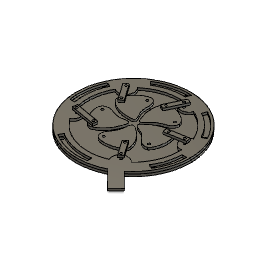
Final Design Machine_Lab v3 (Autodesk Fusion 360 design; units mm, degrees)
Autodesk Fusion 360 part; units mm, degrees
note: some values were not read from the file. Chosen so that the rebuilt part matches the saved one: which face or edge a step refers to; which pieces of a blend or face edit are solid. Set by a fixed rule: which sketch regions a step uses.
sketch "Sketch1" plane through (0, 0, 0) normal (0, 1, 0) x (1, 0, 0)
  spline S0 degree 5 poles (43.1472, 9.785) (42.8335, 10.0513) (42.2447, 10.6075) (41.4786, 11.5091) (40.6873, 12.8271) (40.039, 14.6039) (39.669, 16.4398) (39.5104, 18.2683) (39.5055, 20.0358) (39.6219, 21.7131) (39.8483, 23.293) (40.1848, 24.7857) (40.6367, 26.2147) (41.2054, 27.6126) (41.8835, 29.017) (42.6573, 30.4642) (43.5081, 31.9837) (44.4141, 33.5928) (45.3515, 35.2894) (46.2961, 37.0569) (47.2231, 38.8737) (48.108, 40.7214) (48.9268, 42.5931) (49.6569, 44.5023) (50.2774, 46.4894) (50.7734, 48.6052) (51.1395, 50.8969) (51.3829, 53.3942) (51.5282, 56.0937) (51.6195, 58.9468) (51.7265, 61.8397) (51.9365, 64.6078) (52.3382, 67.0688) (53.0087, 69.0486) (53.9988, 70.4124) (55.3203, 71.0893) (56.9281, 71.1087) (58.7211, 70.6031) (60.5747, 69.7568) (62.3681, 68.7656) (64.0107, 67.796) (65.4747, 66.9355) (66.8035, 66.1769) (68.0742, 65.4622) (69.3697, 64.7133) (70.7494, 63.8669) (72.2158, 62.9108) (73.7306, 61.8713) (75.2356, 60.7928) (76.6724, 59.7206) (78.0017, 58.683) (79.2251, 57.6714) (80.3713, 56.6546) (81.4803, 55.5943) (82.5892, 54.4597) (83.7144, 53.2457) (84.8468, 51.9761) (85.9638, 50.6877) (87.0375, 49.4184) (88.0438, 48.1947) (88.9725, 47.0168) (89.8262, 45.864) (90.615, 44.7065) (91.3529, 43.5148) (92.0529, 42.2719) (92.7251, 40.9743) (93.3772, 39.6256) (94.0137, 38.2321) (94.6358, 36.797) (95.2405, 35.3195) (95.8174, 33.7994) (96.346, 32.2408) (96.7937, 30.6562) (97.1124, 29.0703) (97.2497, 27.5139) (97.1612, 26.017) (96.8208, 24.6027) (96.2362, 23.2791) (95.4444, 22.0397) (94.4944, 20.8698) (93.4345, 19.752) (92.2942, 18.6713) (91.0807, 17.6187) (89.7888, 16.5895) (88.4086, 15.5838) (86.9335, 14.6055) (85.3692, 13.6624) (83.7312, 12.7642) (82.0403, 11.9209) (80.3194, 11.1409) (78.5894, 10.4292) (76.8652, 9.7847) (75.1538, 9.2021) (73.4537, 8.6732) (71.7531, 8.1897) (70.03, 7.7448) (68.2496, 7.336) (66.369, 6.9655) (64.3477, 6.6411) (62.1551, 6.3764) (59.781, 6.1914) (57.2425, 6.1123) (54.5961, 6.1733) (51.9277, 6.4117) (49.3395, 6.8633) (46.9368, 7.5572) (45.2398, 8.3201) (44.1268, 9.0096) (43.4609, 9.5186) (43.1472, 9.785) knots 0 0 0 0 0 0 0.00952381 0.01904762 0.02857143 0.03809524 0.04761905 0.05714286 0.06666667 0.07619048 0.08571429 0.0952381 0.1047619 0.11428571 0.12380952 0.13333333 0.14285714 0.15238095 0.16190476 0.17142857 0.18095238 0.19047619 0.2 0.20952381 0.21904762 0.22857143 0.23809524 0.24761905 0.25714286 0.26666667 0.27619048 0.28571429 0.2952381 0.3047619 0.31428571 0.32380952 0.33333333 0.34285714 0.35238095 0.36190476 0.37142857 0.38095238 0.39047619 0.4 0.40952381 0.41904762 0.42857143 0.43809524 0.44761905 0.45714286 0.46666667 0.47619048 0.48571429 0.4952381 0.5047619 0.51428571 0.52380952 0.53333333 0.54285714 0.55238095 0.56190476 0.57142857 0.58095238 0.59047619 0.6 0.60952381 0.61904762 0.62857143 0.63809524 0.64761905 0.65714286 0.66666667 0.67619048 0.68571429 0.6952381 0.7047619 0.71428571 0.72380952 0.73333333 0.74285714 0.75238095 0.76190476 0.77142857 0.78095238 0.79047619 0.8 0.80952381 0.81904762 0.82857143 0.83809524 0.84761905 0.85714286 0.86666667 0.87619048 0.88571429 0.8952381 0.9047619 0.91428571 0.92380952 0.93333333 0.94285714 0.95238095 0.96190476 0.97142857 0.98095238 0.99047619 1 1 1 1 1 1
  circle A0 centre (87.7815, 27.0791) radius 2.5
  circle A1 centre (49.0696, 16.7654) radius 2.5
  point P0 (39.5371, 18.5455)
  point P1 (40.5207, 25.7886)
  point P2 (43.7661, 32.4418)
  point P3 (48.7966, 42.3405)
  point P4 (51.5553, 57.1074)
  point P5 (54.86, 70.745)
  point P6 (63.3741, 68.1694)
  point P7 (69.5405, 64.5993)
  point P8 (76.7468, 59.6518)
  point P9 (82.1013, 54.9504)
  point P10 (87.2751, 49.1235)
  point P11 (90.9055, 44.2224)
  point P12 (93.7191, 38.8675)
  point P13 (96.3512, 32.1512)
  point P14 (96.9865, 25.4349)
  point P15 (93.9006, 20.2615)
  point P16 (88.1827, 15.4511)
  point P17 (79.7419, 10.9131)
  point P18 (71.0288, 8.0087)
  point P19 (59.2299, 6.1935)
  dimension "d3" = 5
  dimension "d4" = 5
  measures "d3" diameter of A0
  measures "d4" diameter of A1
extrude "Extrude1" add sketch "Sketch1" along normal blind 5 makes body 1
copy_body "CopyPasteBodies1" bodies 1 makes body 2
move_body "Move1" bodies 2 to x (0.34202, 0, -0.939693) y (0, 1, 0) z (0.939693, 0, 0.34202) at (102.3883, 0, -0.091)
copy_body "CopyPasteBodies2" bodies 1 makes body 3
move_body "Move2" bodies 3 to x (-0.766044, 0, -0.642788) y (0, 1, 0) z (0.642788, 0, -0.766044) at (136.402, 0, -96.2286)
copy_body "CopyPasteBodies3" bodies 1 makes body 4
move_body "Move3" bodies 4 to x (-0.866025, 0, 0.5) y (0, 1, 0) z (-0.5, 0, -0.866025) at (56.8274, 0, -161.7752)
copy_body "CopyPasteBodies4" bodies 1 makes body 5
move_body "Move4" bodies 5 to x (0.258819, 0, 0.965926) y (0, 1, 0) z (-0.965926, 0, 0.258819) at (-32.6183, 0, -104.1545)
move_body "Move5" bodies 1 to x (1, 0, 0) y (0, 1, 0) z (0, 0, 1) at (0.8483, 0, 2.8278)
move_body "Move6" bodies 2 to x (1, 0, 0) y (0, 1, 0) z (0, 0, 1) at (1.9795, 0, 1.4139)
move_body "Move7" bodies 3 to x (1, 0, 0) y (0, 1, 0) z (0, 0, 1) at (2.2623, 0, -1.6967)
move_body "Move8" bodies 4 to x (1, 0, 0) y (0, 1, 0) z (0, 0, 1) at (-0.2828, 0, -2.2623)
sketch "Sketch2" plane through (0, 0, 0) normal (0, 1, 0) x (1, 0, 0)
  line L0 (139.8204, 345.519) -> (149.2644, 342.0971)
  line L1 (130.3036, 273.8084) -> (140.4716, 273.8084)
  line L2 (265.593, 175.8364) -> (265.593, 185.9491)
  line L3 (183.8365, 193.5151) -> (188.7923, 202.2173)
  line L4 (341.7338, 236.2587) -> (350.5894, 231.5629)
  line L5 (358.4328, 291.1667) -> (368.4373, 291.1667)
  line L6 (301.1109, 391.2064) -> (304.896, 400.5259)
  line L7 (346.1616, 345.2035) -> (355.4143, 349.0764)
  line L8 (190.9901, 388.388) -> (184.0867, 395.8662)
  line L9 (251.7841, 404.5614) -> (255.7756, 414.3893)
  arc A0 (160.575, 342.2715) -> (182.2812, 369.5563) centre (170.2298, 356.8672) ccw
  arc A1 (139.8204, 345.519) -> (130.3036, 273.8084) centre (248.4867, 294.6109) ccw
  arc A2 (149.2644, 342.0971) -> (140.4716, 273.8084) centre (248.4867, 294.6109) ccw
  arc A3 (166.7528, 236.9952) -> (151.9401, 268.5579) centre (157.9603, 252.126) ccw
  arc A4 (188.7923, 202.2173) -> (265.593, 185.9491) centre (248.4867, 294.6109) ccw
  arc A5 (316.5154, 221.3163) -> (287.2171, 202.4157) centre (302.6963, 210.5792) ccw
  arc A6 (183.8365, 193.5151) -> (265.593, 175.8364) centre (248.4867, 294.6109) ccw
  arc A7 (340.505, 333.7598) -> (348.3504, 299.8302) centre (346.1313, 317.1889) ccw
  arc A8 (341.7338, 236.2587) -> (358.4328, 291.1667) centre (248.4867, 294.6109) ccw
  arc A9 (350.5894, 231.5629) -> (368.4373, 291.1667) centre (248.4867, 294.6109) ccw
  arc A10 (355.4143, 349.0764) -> (304.896, 400.5259) centre (248.4867, 294.6109) ccw
  arc A11 (255.7756, 414.3893) -> (184.0867, 395.8662) centre (248.4867, 294.6109) ccw
  arc A12 (255.2403, 394.3826) -> (289.0833, 385.9997) centre (272.5299, 391.6775) ccw
  arc A13 (346.1616, 345.2035) -> (301.1109, 391.2064) centre (248.4867, 294.6109) ccw
  arc A14 (251.7841, 404.5614) -> (190.9901, 388.388) centre (248.4867, 294.6109) ccw
  circle A15 centre (270.502, 383.7695) radius 2.5
  circle A16 centre (175.5823, 351.1974) radius 2.5
  circle A17 centre (163.4194, 255.7635) radius 2.5
  circle A18 centre (298.976, 216.8085) radius 2.5
  circle A19 centre (340.3926, 315.4967) radius 2.5
  arc A20 (160.575, 342.2715) -> (151.9401, 268.5579) centre (248.4867, 294.6109) ccw
  arc A21 (166.7528, 236.9952) -> (287.2171, 202.4157) centre (248.4867, 294.6109) ccw
  arc A22 (316.5154, 221.3163) -> (348.3504, 299.8302) centre (248.4867, 294.6109) ccw
  arc A23 (340.505, 333.7598) -> (289.0833, 385.9997) centre (248.4867, 294.6109) ccw
  arc A24 (255.2403, 394.3826) -> (182.2812, 369.5563) centre (248.4867, 294.6109) ccw
  line L10 (326.1265, 196.6462) -> (358.946, 163.8249)
  line L11 (358.946, 163.8249) -> (340.1469, 145.7773)
  line L12 (340.1469, 145.7773) -> (304.4024, 182.8145)
  arc A25 (326.1265, 196.6462) -> (304.4024, 182.8145) centre (248.4867, 294.6109) ccw
  dimension "d7" = 250
  dimension "d9" = 200
  dimension "d11" = 35
  dimension "d13" = 35
  dimension "d14" = 35
  dimension "d15" = 35
  dimension "d16" = 35
  dimension "d21" = 240
  dimension "d22" = 220
  dimension "d23" = 5
  dimension "d24" = 5
  dimension "d25" = 5
  dimension "d26" = 5
  dimension "d27" = 5
  constraint coincident A1.centre A2.centre
  constraint coincident A5.centre A20
  constraint coincident A3.centre A20
  constraint coincident A12.centre A20
  constraint coincident A0.centre A20
  constraint concentric A1 A2
  constraint horizontal L1
  constraint coincident L2.start A1
  constraint coincident L2.end A2
  constraint perpendicular L1 L2
  constraint coincident L3.start A1
  constraint coincident L3.end A2
  constraint coincident L4.start A2
  constraint coincident L4.end A1
  constraint coincident L5.start A2
  constraint coincident L5.end A1
  constraint horizontal L5
  constraint coincident L6.start A2
  constraint coincident L6.end A1
  constraint coincident L7.start A2
  constraint coincident L7.end A1
  constraint coincident L9.start A2
  constraint coincident L9.end A1
  constraint parallel L6 L9
  constraint concentric A1 A6
  constraint concentric A2 A4
  constraint coincident A3.start A20
  constraint concentric A4 A8
  constraint coincident A5.end A20
  constraint coincident A5.start A20
  constraint concentric A6 A9
  constraint coincident A7.start A20
  constraint concentric A8 A13
  constraint concentric A9 A10
  constraint coincident A7.end A20
  constraint concentric A10 A11
  constraint concentric A13 A14
  constraint coincident A12.end A20
  constraint coincident A12.start A20
  constraint concentric A20 A21
  constraint concentric A21 A22
  constraint concentric A22 A23
  constraint concentric A23 A24
  measures "d7" diameter of A25
  measures "d9" diameter of A20
  measures "d11" diameter of A5
  measures "d13" diameter of A3
  measures "d14" diameter of A0
  measures "d15" diameter of A12
  measures "d16" diameter of A7
  measures "d21" diameter of A1
  measures "d22" diameter of A2
  measures "d23" diameter of A15
  measures "d24" diameter of A16
  measures "d25" diameter of A17
  measures "d26" diameter of A18
  measures "d27" diameter of A19
extrude "Extrude2" add sketch "Sketch2" along normal blind 5 separate body makes body 6
move_body "Move9" bodies 2 1 4 3 5 to x (1, 0, 0) y (0, 1, 0) z (0, 0, 1) at (196.2981, 0, -221.2248)
move_body "Move10" bodies 1 2 5 3 4 to x (1, 0, 0) y (0, 1, 0) z (0, 0, 1) at (-240.9487, 0, 32.4034)
move_body "Move11" bodies 3 to x (0.34202, 0, -0.939693) y (0, 1, 0) z (0.939693, 0, 0.34202) at (499.9705, 0, -200.872)
move_body "Move12" bodies 2 to x (0.34202, 0, -0.939693) y (0, 1, 0) z (0.939693, 0, 0.34202) at (503.687, 0, -198.4468)
move_body "Move13" bodies 3 2 to x (1, 0, 0) y (0, 1, 0) z (0, 0, 1) at (-3.7389, 0, 0)
move_body "Move14" bodies 4 to x (-0.766044, 0, 0.642788) y (0, 1, 0) z (-0.642788, 0, -0.766044) at (90.3797, 0, -493.662)
move_body "Move15" bodies 1 to x (0.173648, 0, 0.984808) y (0, 1, 0) z (-0.984808, 0, 0.173648) at (-8.1527, 0, -252.2029)
move_body "Move16" bodies 5 to x (0.34202, 0, -0.939693) y (0, 1, 0) z (0.939693, 0, 0.34202) at (496.7531, 0, -192.5985)
move_body "Move28" bodies 2 to x (1, 0, 0) y (0, 1, 0) z (0, 0, 1) at (0, 5, 0)
move_body "Move29" bodies 3 to x (1, 0, 0) y (0, 1, 0) z (0, 0, 1) at (0, 5, 0)
move_body "Move30" bodies 1 to x (1, 0, 0) y (0, 1, 0) z (0, 0, 1) at (0, 5, 0)
move_body "Move31" bodies 5 to x (1, 0, 0) y (0, 1, 0) z (0, 0, 1) at (0, 5, 0)
move_body "Move32" bodies 4 to x (1, 0, 0) y (0, 1, 0) z (0, 0, 1) at (0, 5, 0)
move_body "Move17" bodies 2 4 3 5 1 to x (1, 0, 0) y (0, 1, 0) z (0, 0, 1) at (-2.4926, 0, -2.908)
sketch "Sketch4" plane through (0, 0, 0) normal (0, 1, 0) x (1, 0, 0)
  circle A0 centre (248.2873, 294.4666) radius 125
  circle A1 centre (348.3605, 238.1051) radius 4
  circle A2 centre (347.9665, 352.0493) radius 4
  circle A3 centre (247.8847, 409.4834) radius 4
  circle A4 centre (190.6001, 195.2892) radius 4
  circle A5 centre (142.3249, 338.8584) radius 4
  circle A6 through (4.5972, 368.5991, 0) (-2.2986, 368.5991, 3.9813) (-2.2986, 368.5991, -3.9813)
  circle A7 centre (163.3113, 255.8537) radius 2.5
  circle A8 centre (175.5685, 351.3554) radius 2.5
  circle A9 centre (270.4135, 383.9297) radius 2.5
  circle A10 centre (340.3533, 315.4907) radius 2.5
  circle A11 centre (298.9335, 216.923) radius 2.5
  circle A12 centre (306.6377, 270.508) radius 2.5
  circle A13 centre (190.0245, 285.0655) radius 2.5
  circle A14 centre (242.9626, 235.5716) radius 2.5
  circle A15 centre (293.3741, 340.3662) radius 2.5
  circle A16 centre (222.4062, 351.2026) radius 2.5
  dimension "d34" = 250
  dimension "d35" = 8
  dimension "d38" = 5
  dimension "d39" = 5
  dimension "d40" = 5
  dimension "d41" = 5
  dimension "d42" = 5
  dimension "d86" = 5
  constraint equal A2 A4
  constraint equal A1 A4
  constraint equal A1 A5
  constraint equal A3 A5
  constraint equal A12 A16
  constraint equal A12 A15
  constraint equal A13 A15
  constraint equal A13 A14
  measures "d34" diameter of A0
  measures "d35" diameter of A1
  measures "d38" diameter of A7
  measures "d39" diameter of A8
  measures "d40" diameter of A9
  measures "d41" diameter of A10
  measures "d42" diameter of A11
  measures "d86" diameter of A12
extrude "Extrude15" add sketch "Sketch4" against normal blind 5 bodies 6
extrude "Extrude14" add sketch "Sketch4" against normal blind 5 contours A0 | A12 | A13 | A14 | A15 | A16 bodies 6
move_body "Move19" bodies 6 1 3 2 4 5 to x (1, 0, 0) y (0, 1, 0) z (0, 0, 1) at (0, 5, 0)
extrude "Extrude3" add sketch "Sketch4" along normal blind 5 bodies 1 2 3 4 5 6
move_body "Move18" bodies 2 5 1 3 6 4 to x (1, 0, 0) y (0, 1, 0) z (0, 0, 1) at (0, 5, 0)
sketch "Sketch3" plane through (0, 0, 0) normal (0, 1, 0) x (1, 0, 0)
sketch "Sketch5" plane through (0, 0, 0) normal (0, 1, 0) x (1, 0, 0)
  line L0 (283.1844, 249.0311) -> (306.1274, 216.265)
  line L1 (306.1274, 216.265) -> (297.9359, 210.5292)
  line L2 (297.9359, 210.5292) -> (274.9929, 243.2953)
  line L3 (274.9929, 243.2953) -> (283.1844, 249.0311)
  circle A0 centre (282.3244, 242.2662) radius 2.5
  circle A1 centre (299.0242, 216.8657) radius 2.5
  dimension "d45" = 10
  dimension "d46" = 40
  dimension "d47" = 5
  dimension "d48" = 5
  measures "d45" distance of L0.start L2.end
  measures "d46" distance of L0.start L0.end
  measures "d47" diameter of A0
  measures "d48" diameter of A1
extrude "Extrude4" add sketch "Sketch5" along normal blind 5 separate body makes body 7
move_body "Move20" bodies 7 to x (1, 0, 0) y (0, 1, 0) z (0, 0, 1) at (0, 40, 0)
sketch "Sketch6" plane through (0, 0, 0) normal (0, 1, 0) x (1, 0, 0)
  line L0 (158.7818, 261.8213) -> (157.0453, 251.9732)
  line L1 (157.0453, 251.9732) -> (211.0329, 242.4537)
  line L2 (211.0329, 242.4537) -> (212.9454, 252.266)
  line L3 (212.9454, 252.266) -> (158.7818, 261.8213)
  circle A0 centre (163.2414, 255.8665) radius 2.5
  circle A1 centre (206.6788, 248.8035) radius 2.5
  dimension "d51" = 10
  dimension "d52" = 55
  dimension "d53" = 5
  constraint equal A0 A1
  measures "d51" distance of L0.start L0.end
  measures "d52" distance of L0.start L2.end
  measures "d53" diameter of A0
extrude "Extrude5" add sketch "Sketch6" along normal blind 5 separate body makes body 8
move_body "Move21" bodies 8 to x (1, 0, 0) y (0, 1, 0) z (0, 0, 1) at (0, 40, 0)
sketch "Sketch7" plane through (0, 0, 0) normal (0, 1, 0) x (1, 0, 0)
  line L0 (193.6109, 315.3858) -> (201.8024, 321.1216)
  line L1 (201.8024, 321.1216) -> (175.9922, 357.9839)
  line L2 (175.9922, 357.9839) -> (167.6295, 352.4911)
  line L3 (167.6295, 352.4911) -> (193.6109, 315.3858)
  circle A0 centre (193.9142, 322.9166) radius 2.5
  circle A1 centre (175.6232, 351.037) radius 2.5
  dimension "d56" = 10
  dimension "d57" = 45
  dimension "d58" = 5
  constraint equal A0 A1
  measures "d56" distance of L0.start L0.end
  measures "d57" distance of L0.end L1.end
  measures "d58" diameter of A0
extrude "Extrude6" add sketch "Sketch7" along normal blind 5 separate body makes body 9
move_body "Move22" bodies 9 to x (1, 0, 0) y (0, 1, 0) z (0, 0, 1) at (0, 40, 0)
sketch "Sketch8" plane through (0, 0, 0) normal (0, 1, 0) x (1, 0, 0)
  line L0 (278.1905, 389.1192) -> (259.1727, 348.3353)
  line L1 (259.1727, 348.3353) -> (249.8769, 352.0625)
  line L2 (249.8769, 352.0625) -> (269.1274, 393.3453)
  line L3 (269.1274, 393.3453) -> (278.1905, 389.1192)
  circle A0 centre (257.2705, 357.2368) radius 2.5
  circle A1 centre (270.5367, 383.6541) radius 2.5
  dimension "d61" = 10
  dimension "d62" = 45
  dimension "d63" = 5
  constraint equal A0 A1
  measures "d61" distance of L0.start L2.end
  measures "d62" distance of L0.start L0.end
  measures "d63" diameter of A0
extrude "Extrude7" add sketch "Sketch8" along normal blind 5 separate body makes body 10
move_body "Move23" bodies 10 to x (1, 0, 0) y (0, 1, 0) z (0, 0, 1) at (0, 40, 0)
sketch "Sketch9" plane through (0, 0, 0) normal (0, 1, 0) x (1, 0, 0)
  line L0 (301.6314, 313.7988) -> (346.1412, 321.6471)
  line L1 (346.1412, 321.6471) -> (347.8777, 311.799)
  line L2 (347.8777, 311.799) -> (303.5614, 303.9848)
  line L3 (303.5614, 303.9848) -> (301.6314, 313.7988)
  circle A0 centre (340.4695, 315.3503) radius 2.5
  circle A1 centre (310.2675, 310.2113) radius 2.5
  dimension "d66" = 10
  dimension "d67" = 45
  dimension "d68" = 5
  constraint equal A0 A1
  measures "d66" distance of L0.end L1.end
  measures "d67" distance of L1.end L2.end
  measures "d68" diameter of A0
extrude "Extrude8" add sketch "Sketch9" along normal blind 5 separate body makes body 11
move_body "Move24" bodies 11 to x (1, 0, 0) y (0, 1, 0) z (0, 0, 1) at (0, 40, 0)
move_body "Move33" bodies 7 10 9 8 11 to x (1, 0, 0) y (0, 1, 0) z (0, 0, 1) at (0, -20, 0)
delete_face "DeleteFace1" 1 faces at (318.8929, 6.6667, -191.3169) on bodies 6
extrude "Extrude16" add sketch "Sketch4" along normal blind 5 separate body makes body 12
move_body "Move34" bodies 12 to x (1, 0, 0) y (0, 1, 0) z (0, 0, 1) at (0, 5, 0)
equation "screw = 5 mm"
equation "Thickness = 5 mm"
equation "d3 = screw"
equation "d4 = screw"
equation "d5 = Thickness"
equation "d7 = OuterBeltDiameter"
equation "OuterBeltDiameter = 250 mm"
equation "beltThickness = 15 mm"
equation "Length = 10 mm"
equation "Width = 70 mm"
equation "d23 = screw"
equation "d24 = screw"
equation "d25 = screw"
equation "d26 = screw"
equation "d27 = screw"
equation "d28 = Thickness"
equation "d35 = Bolt"
equation "Bolt = 8 mm"
equation "d38 = screw"
equation "d39 = screw"
equation "d40 = screw"
equation "d41 = screw"
equation "d42 = screw"
equation "d43 = Thickness"
equation "d47 = screw"
equation "d48 = screw"
equation "d49 = Thickness"
equation "d53 = screw"
equation "d54 = Thickness"
equation "d58 = screw"
equation "d59 = Thickness"
equation "d63 = screw"
equation "d64 = Thickness"
equation "d68 = screw"
equation "d69 = Thickness"
equation "d84 = -Thickness"
equation "d86 = screw"
equation "d87 = -Thickness"
equation "d89 = Thickness"
